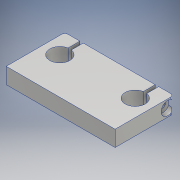
# Autodesk Inventor part: suporte_guia_linear_cabeça_superior
Saved by Autodesk Inventor 2018 (Build 220112000, 112)
## iProperties
Created: 2018-05-17
Part Number: suporte_guia_linear_cabeça_superior
Material: Alumínio 6061
Document SubType Name: Modeling
Designer: Usuario
Density: 2.7 g/cm^3
Appearance: Alumínio - Plano
Author: Usuario
Autodesk Inventor part; units mm, degrees
ref_plane "YZ Plane" through (0, 0, 0) normal (1, 0, 0) x (0, 1, 0)
ref_plane "XZ Plane" through (0, 0, 0) normal (0, 1, 0) x (-1, 0, 0)
ref_plane "XY Plane" through (0, 0, 0) normal (0, 0, 1) x (1, 0, 0)
sketch "Esboço1" plane through (0, 0, 0) normal (0, 0, 1) x (1, 0, 0)
  line L0 (0, 0) -> (-32.5, 0)
  line L1 (-30, 12) -> (-30, 12)
  line L2 (0, 22) -> (-32.5, 22) construction
  arc A0 (-23.5, 27.9161) -> (-21.5, 27.9161) centre (-22.5, 22) ccw
  line L3 (-22.5, 22) -> (-22.5, 35) construction
  line L4 (-21.5, 27.9161) -> (-21.5, 35)
  line L5 (-23.5, 9) -> (-21.5, 35) construction
  line L6 (-21.5, 9) -> (-23.5, 35) construction
  line L7 (-23.5, 35) -> (-23.5, 27.9161)
  line L8 (-21.5, 35) -> (0, 35)
  line L9 (-32.5, 0) -> (-32.5, 33)
  line L10 (-30.5, 35) -> (-23.5, 35)
  arc A1 (-30.5, 35) -> (-32.5, 33) centre (-30.5, 33) ccw
  line L11 (0, 44.6539) -> (0, -19.6488) construction
  line L12 (0, 0) -> (32.5, 0)
  line L13 (30, 12) -> (30, 12)
  line L14 (0, 22) -> (32.5, 22) construction
  arc A2 (21.5, 27.9161) -> (23.5, 27.9161) centre (22.5, 22) ccw
  line L15 (22.5, 22) -> (22.5, 35) construction
  line L16 (21.5, 27.9161) -> (21.5, 35)
  line L17 (23.5, 9) -> (21.5, 35) construction
  line L18 (21.5, 9) -> (23.5, 35) construction
  line L19 (23.5, 35) -> (23.5, 27.9161)
  line L20 (21.5, 35) -> (0, 35)
  line L21 (32.5, 0) -> (32.5, 33)
  line L22 (30.5, 35) -> (23.5, 35)
  arc A3 (32.5, 33) -> (30.5, 35) centre (30.5, 33) ccw
  dimension "d0" = 32.5
  dimension "d16" = 12
  dimension "d24" = 10
  dimension "d25" = 2
  dimension "d26" = 35
  dimension "d27" = 2
  constraints: 46 end point, 15 symmetric about line, 8 point on circle, 4 centre point, 4 midpoint, 2 horizontal, 2 perpendicular, 2 tangent, 2 vertical, 1 parallel, 2 other
  measures "d0" distance of L0.start L0.end
  measures "d16" diameter of A0
  measures "d24" distance of L2.end L3.start
  measures "d25" distance of L6.end L4.end
  measures "d26" distance between parallel lines of L0 L10
  measures "d27" radius of A1
extrude "Extrusão1" add sketch "Esboço1" along normal mid plane 9.5
sketch "Esboço2" plane through (21.5, 27.9161, 4.75) normal (1, 0, 0) x (0, 0, -1)
  circle A0 centre (4.75, 3.542) radius 2
  point P0 (4.75, -27.9161)
  dimension "d31" = 4
  constraints: 1 centre point
  measures "d31" diameter of A0
hole "Furo1" at (21.5, 31.458, 0) direction (-1, 0, 0) diameter 3.242 depth 15 tip angle 118 thread size "M4x0.7" class "6H" standard "ANSI Metric M Profile"
sketch "Esboço3" plane through (-21.5, 27.9161, 4.75) normal (-1, 0, 0) x (0, 0, 1)
  circle A0 centre (-4.75, 3.542) radius 1.621 projected
  circle A1 centre (-4.75, 3.542) radius 2
  point P0 (-4.75, -27.9161)
  dimension "d39" = 4
  constraints: 1 centre point, 1 coincident
  measures "d39" diameter of A1
hole "Furo2" at (-21.5, 31.458, 0) direction (1, 0, 0) diameter 3.242 depth 15 tip angle 118 thread size "M4x0.7" class "6H" standard "ANSI Metric M Profile"
sketch "Esboço4" plane through (-32.5, 0, 4.75) normal (-1, 0, 0) x (0, 0, 1)
  circle A0 centre (-4.75, 31.458) radius 1.621 projected
  circle A1 centre (-4.75, 31.458) radius 1.621
  point P0 (-4.75, 0)
  constraints: 1 centre point, 1 coincident
hole "Furo3" at (-32.5, 31.458, 0) direction (1, 0, 0) diameter 3 end up to face face through (-23.5, 30.2774, 1.5833) facing (1, 0, 0) counterbore diameter 8 counterbore depth 3
sketch "Esboço5" plane through (32.5, 0, 4.75) normal (1, 0, 0) x (0, 0, -1)
  circle A0 centre (4.75, 31.458) radius 1.5 projected
  circle A1 centre (4.75, 31.458) radius 2
  point P0 (4.75, 0)
  dimension "d54" = 4
  constraints: 1 centre point, 1 coincident
  measures "d54" diameter of A1
hole "Furo4" at (32.5, 31.458, 0) direction (-1, 0, 0) diameter 3 end up to face face through (23.5, 32.6387, 1.5833) facing (-1, 0, 0) counterbore diameter 8 counterbore depth 3
